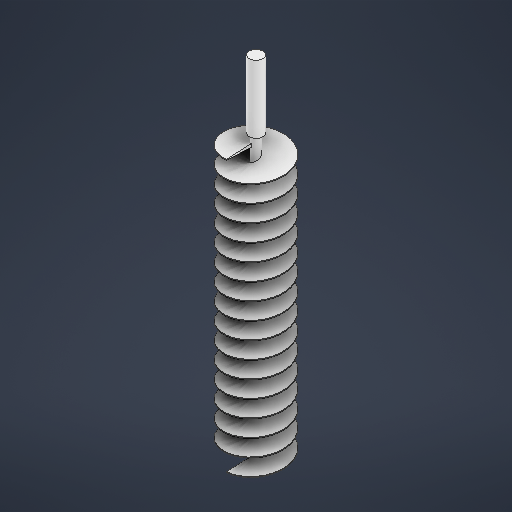
# Autodesk Inventor part: auger
Saved by Autodesk Inventor 2027 (Build 310192060, 192F)
## iProperties
Created: 2026-08-20
Part Number: auger
Material: PVC-Piping
Document SubType Name: Modeling
Designer: trtrn
Density: 1.4 g/cm^3
Appearance: Smooth - White
Author: trtrn
Autodesk Inventor part; units mm, degrees
ref_plane "YZ Plane" through (0, 0, 0) normal (1, 0, 0) x (0, 1, 0)
ref_plane "XZ Plane" through (0, 0, 0) normal (0, 1, 0) x (-1, 0, 0)
ref_plane "XY Plane" through (0, 0, 0) normal (0, 0, 1) x (1, 0, 0)
sketch "Sketch1" plane through (0, 0, 0) normal (0, 1, 0) x (-1, 0, 0)
  circle A0 centre (0, 0) radius 2.5
  dimension "d0" = 5
  constraints: 1 centre point, 1 coincident
  measures "d0" diameter of A0
extrude "Extrusion1" add sketch "Sketch1" along normal blind 166
sketch "Sketch2" plane through (0, 0, 0) normal (1, 0, 0) x (0, 1, 0)
  line L0 (0, 2.5) -> (166, 2.5) projected
  line L1 (0, 2.5) -> (2, 2.5)
  line L2 (2, 2.5) -> (1.25, 17.5)
  line L3 (0.75, 17.5) -> (0, 2.5)
  line L4 (1, 2.5) -> (1, 17.5) construction
  line L5 (0.75, 17.5) -> (1.25, 17.5)
  point P0 (0, 0)
  dimension "d13" = 2
  dimension "d14" = 15
  dimension "d15" = 0.5
  constraints: 10 end point, 2 horizontal, 2 midpoint, 1 vertical, 1 other
  measures "d13" distance of L1.end L0.start
  measures "d14" distance of L4.end L4.start
  measures "d15" distance of L3.start L2.end
coil "Coil1" sketch "Sketch2" operation add axis through (0, -10, 0) along (0, 1, 0) pitch 10 turns 16 hand right
sketch "Sketch3" plane through (0, 166, 0) normal (0, 1, 0) x (1, 0, 0)
  circle A0 centre (0, 0) radius 4
  circle A1 centre (0, 0) radius 2.5 projected
  dimension "d18" = 8
  constraints: 1 centre point, 1 coincident, 1 concentric
  measures "d18" diameter of A0
extrude "Extrusion2" add sketch "Sketch3" along normal blind 40 contours A0 | A1
body "Solid1"
